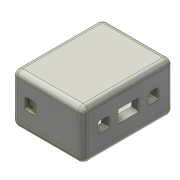
# Autodesk Inventor part: корпус емкость
Saved by Autodesk Inventor 2021 (Build 250183000, 183)
## iProperties
Created: 2023-02-13
Part Number: корпус емкость
Material: Типовые
Document SubType Name: Modeling
Designer: Tasya
Density: 1 g/cm^3
Appearance: Гладкий - слоновая кость
Author: Tasya
Autodesk Inventor part; units mm, degrees
ref_plane "YZ Plane" through (0, 0, 0) normal (1, 0, 0) x (0, 1, 0)
ref_plane "XZ Plane" through (0, 0, 0) normal (0, 1, 0) x (-1, 0, 0)
sketch "Эскиз1" plane through (0, 0, 0) normal (0, 1, 0) x (-1, 0, 0)
  line L0 (-20, 30) -> (20, 30)
  line L1 (20, 30) -> (20, -30)
  line L2 (20, -30) -> (-20, -30)
  line L3 (-20, -30) -> (-20, 30)
  line L4 (-20, 30) -> (20, -30) construction
  line L5 (20, 30) -> (-20, -30) construction
  point P0 (0, 0)
  dimension "d0" = 40
  dimension "d1" = 60
  constraints: 12 end point, 2 midpoint, 2 parallel, 1 horizontal, 1 perpendicular
  measures "d0" distance of L1.end L2.end
  measures "d1" distance of L0.end L1.end
extrude "Выдавливание1" add sketch "Эскиз1" along normal blind 30
shell "Оболочка1" thickness 3 outward yes removed faces 0
sketch "Эскиз22" plane through (-23, 0, -30) normal (1, 0, 0) x (0, 0, -1)
  line L0 (0, 0) -> (-60, 0) projected
  line L1 (0, 0) -> (0, 30) projected
  line L2 (0, 30) -> (-60, 30) projected
  line L3 (-60, 0) -> (-60, 30) projected
  line L4 (3, -3) -> (-63, -3) projected
  line L5 (-63, -3) -> (-63, 33) projected
  line L6 (3, 33) -> (-63, 33) projected
  line L7 (3, -3) -> (3, 33) projected
extrude "Выдавливание15" add sketch "Эскиз22" against normal blind 3 contours L0 L3 L2 L1 | L4 L5 L6 L7
sketch "Эскиз23" plane through (23, 0, 30) normal (-1, 0, 0) x (0, 0, 1)
  line L0 (0, 0) -> (-60, 0) projected
  line L1 (0, 0) -> (0, 30) projected
  line L2 (0, 30) -> (-60, 30) projected
  line L3 (-60, 0) -> (-60, 30) projected
  line L4 (3, -3) -> (-63, -3) projected
  line L5 (-63, -3) -> (-63, 33) projected
  line L6 (3, 33) -> (-63, 33) projected
  line L7 (3, -3) -> (3, 33) projected
  point P0 (-30, 0)
extrude "Выдавливание16" add sketch "Эскиз23" against normal blind 3 contours L0 L3 L2 L1 | L4 L5 L6 L7
fillet "Сопряжение1" radius 4 12 edges at (0, 33, 33) (0, -3, 33) (0, 33, -33) (0, -3, -33) (-26, 15, 33) (-26, 33, 0) (-26, -3, 0) (-26, 15, -33) (26, -3, 0) (26, 15, -33) (26, 33, 0) (26, 15, 33)
ref_plane "РабПлоскость1" through (0, 3, 0) normal (0, -1, 0) x (1, 0, 0)
split body "Разделение1" result two bodies by plane through (0, 3, 0) normal (0, -1, 0) first body at (7.333333, -2.5, 9.666667)
sketch "Эскиз24" plane through (-26, 3, 33) normal (0, -1, 0) x (1, 0, 0)
  line L0 (46, -63) -> (6, -63) construction
  line L1 (46, -3) -> (46, -63) construction
  line L2 (6, -3) -> (46, -3) construction
  line L3 (6, -63) -> (6, -3) construction
  line L4 (49, -3) -> (49, -63) construction
  line L5 (49, -63) -> (3, -63) construction
  line L6 (3, -63) -> (3, -3) construction
  line L7 (3, -3) -> (49, -3) construction
  line L8 (49, -3) -> (3, -63) construction
  line L9 (49, -63) -> (3, -3) construction
  line L10 (3, -3) -> (8, -8) construction
  line L11 (3, -3) -> (10.071068, -3) construction
  circle A0 centre (5.5, -5.5) radius 1.85 construction
  circle A1 centre (5.5, -5.5) radius 3.535534
  circle A2 centre (46.5, -5.5) radius 3.535534
  circle A3 centre (5.5, -60.5) radius 3.535534
  circle A4 centre (46.5, -60.5) radius 3.535534
  point P0 (26, -33)
  point P1 (44, -3)
  point P2 (3, -58)
  point P3 (44, -58)
  dimension "d168" = 45
  dimension "d169" = 3.7
  dimension "d170" = 2.5
  dimension "d171" = 46
  dimension "d172" = 60
  dimension "d175" = 41
  dimension "d178" = 55
  dimension "d230" = 3
  constraints: 16 end point, 3 horizontal, 3 midpoint, 3 vertical, 2 parallel, 1 centre point, 1 coincident, 1 collinear, 1 equal length, 1 perpendicular, 18 other
  measures "d168" angle of L10 L11
  measures "d169" diameter of A0
  measures "d170" distance from line of L2 A0.centre
  measures "d171" distance between parallel lines of L4 L6
  measures "d172" distance of L4.start L4.end
  measures "d175" distance of point (5.5, -5.5) point (46.5, -5.5)
  measures "d178" distance of point (5.5, -5.5) point (5.5, -60.5)
  measures "d230" distance between parallel lines of L4 L1
extrude "Выдавливание17" add sketch "Эскиз24" against normal up to next bodies 3
fillet "Сопряжение2" radius 2 16 edges at (-20, 30, 0) (0, 30, -30) (20, 30, 0) (0, 30, 30) (17.1459, 30, 26.382) (18, 16.5, 30) (20, 16.5, 24) (-20, 16.5, 24) (-18, 16.5, 30) (-17.1459, 30, 26.382) (-20, 16.5, -24) (-17.1459, 30, -26.382) (-18, 16.5, -30) (17.1459, 30, -26.382) (20, 16.5, -24) (18, 16.5, -30)
sketch "Эскиз25" plane through (-26, 3, 33) normal (0, -1, 0) x (1, 0, 0)
  line L0 (52, -4) -> (52, -62)
  line L1 (4, 0) -> (48, 0)
  line L2 (0, -62) -> (0, -4)
  line L3 (48, -66) -> (4, -66)
  arc A0 (7.096745, -8.654426) -> (9.021082, -5.180651) centre (5.5, -5.5) ccw
  line L4 (40.987094, -3) -> (11.012906, -3)
  arc A1 (42.978918, -5.180651) -> (44.903255, -8.654426) centre (46.5, -5.5) ccw
  arc A2 (46, -10.43884) -> (44.903255, -8.654426) centre (44, -10.43884) ccw
  line L5 (46, -55.56116) -> (46, -10.43884)
  arc A3 (44.903255, -57.345574) -> (46, -55.56116) centre (44, -55.56116) ccw
  arc A4 (44.903255, -57.345574) -> (42.978918, -60.819349) centre (46.5, -60.5) ccw
  line L6 (11.012906, -63) -> (40.987094, -63)
  arc A5 (9.021082, -60.819349) -> (7.096745, -57.345574) centre (5.5, -60.5) ccw
  arc A6 (6, -55.56116) -> (7.096745, -57.345574) centre (8, -55.56116) ccw
  line L7 (6, -10.43884) -> (6, -55.56116)
  arc A7 (7.096745, -8.654426) -> (6, -10.43884) centre (8, -10.43884) ccw
  arc A8 (0, -62) -> (4, -66) centre (4, -62) ccw
  arc A9 (48, -66) -> (52, -62) centre (48, -62) ccw
  arc A10 (52, -4) -> (48, 0) centre (48, -4) ccw
  arc A11 (4, 0) -> (0, -4) centre (4, -4) ccw
  arc A12 (11.012906, -3) -> (9.021082, -5.180651) centre (11.012906, -5) ccw
  arc A13 (42.978918, -5.180651) -> (40.987094, -3) centre (40.987094, -5) ccw
  arc A14 (40.987094, -63) -> (42.978918, -60.819349) centre (40.987094, -61) ccw
  arc A15 (9.021082, -60.819349) -> (11.012906, -63) centre (11.012906, -61) ccw
  point P0 (26, -33)
  point P1 (5.5, -5.5)
  point P2 (5.5, -60.5)
  constraints: 4 coincident
hole "Отверстие5" at (-20.5, 3, 27.5) at (20.5, 3, 27.5) at (-20.5, 3, -27.5) at (20.5, 3, -27.5) direction (0, 1, 0) diameter 3.7 depth 6 countersink diameter 4 countersink angle 90 bodies 3
sketch "Эскиз26" plane through (-26, 3, -33) normal (0, 1, 0) x (1, 0, 0)
  circle A0 centre (5.5, -5.5) radius 2
  circle A1 centre (5.5, -60.5) radius 2
  circle A2 centre (46.5, -60.5) radius 2
  circle A3 centre (46.5, -5.5) radius 2
  line L0 (52, -62) -> (52, -4)
  line L1 (4, -66) -> (48, -66)
  line L2 (0, -4) -> (0, -62)
  line L3 (48, 0) -> (4, 0)
  arc A4 (9.021082, -60.819349) -> (7.096745, -57.345574) centre (5.5, -60.5) ccw
  line L4 (40.987094, -63) -> (11.012906, -63)
  arc A5 (44.903255, -57.345574) -> (42.978918, -60.819349) centre (46.5, -60.5) ccw
  arc A6 (44.903255, -57.345574) -> (46, -55.56116) centre (44, -55.56116) ccw
  line L5 (46, -10.43884) -> (46, -55.56116)
  arc A7 (46, -10.43884) -> (44.903255, -8.654426) centre (44, -10.43884) ccw
  arc A8 (42.978918, -5.180651) -> (44.903255, -8.654426) centre (46.5, -5.5) ccw
  line L6 (11.012906, -3) -> (40.987094, -3)
  arc A9 (7.096745, -8.654426) -> (9.021082, -5.180651) centre (5.5, -5.5) ccw
  arc A10 (7.096745, -8.654426) -> (6, -10.43884) centre (8, -10.43884) ccw
  line L7 (6, -55.56116) -> (6, -10.43884)
  arc A11 (6, -55.56116) -> (7.096745, -57.345574) centre (8, -55.56116) ccw
  arc A12 (4, 0) -> (0, -4) centre (4, -4) ccw
  arc A13 (52, -4) -> (48, 0) centre (48, -4) ccw
  arc A14 (48, -66) -> (52, -62) centre (48, -62) ccw
  arc A15 (0, -62) -> (4, -66) centre (4, -62) ccw
  arc A16 (9.021082, -60.819349) -> (11.012906, -63) centre (11.012906, -61) ccw
  arc A17 (40.987094, -63) -> (42.978918, -60.819349) centre (40.987094, -61) ccw
  arc A18 (42.978918, -5.180651) -> (40.987094, -3) centre (40.987094, -5) ccw
  arc A19 (11.012906, -3) -> (9.021082, -5.180651) centre (11.012906, -5) ccw
  point P0 (26, -33)
extrude "Выдавливание18" add sketch "Эскиз26" against normal up to next contours A0 | A1 | A2 | A3 | A14 L1 A15 L2 A12 L3 A13 L0 bodies 2
fillet "Сопряжение3" radius 2 12 edges at (-20, 0, 0) (0, 0, 30) (19.7039, 0, 23.6084) (20, 0, 0) (19.7039, 0, -23.6084) (17.4073, 0, -25.7868) (17.4073, 0, 25.7868) (0, 0, -30) (-19.7039, 0, 23.6084) (-17.4073, 0, 25.7868) (-19.7039, 0, -23.6084) (-17.4073, 0, -25.7868)
sketch "Эскиз28" plane through (26, 0, 30) normal (1, 0, 0) x (0, 0, -1)
  line L0 (1, 3) -> (59, 3) projected
  line L1 (59, 29) -> (59, 3) projected
  line L2 (1, 29) -> (59, 29) projected
  line L3 (1, 3) -> (1, 29) projected
  line L4 (22.6, 20.5) -> (37.4, 20.5)
  line L5 (37.4, 20.5) -> (37.4, 11.5)
  line L6 (37.4, 11.5) -> (22.6, 11.5)
  line L7 (22.6, 11.5) -> (22.6, 20.5)
  line L8 (22.6, 20.5) -> (37.4, 11.5) construction
  line L9 (37.4, 20.5) -> (22.6, 11.5) construction
  line L10 (30, 0) -> (30, -11) construction
  line L11 (1, 3) -> (1, 29) construction
  line L12 (1, 16) -> (7, 16) construction
  point P0 (30, 16)
  point P1 (30, 16)
  point P2 (30, 16)
  dimension "d199" = 9
  dimension "d200" = 14.8
  constraints: 16 end point, 5 midpoint, 2 horizontal, 2 parallel, 2 point on line, 1 perpendicular, 1 vertical
  measures "d199" distance of L6.end L4.start
  measures "d200" distance of L5.end L6.end
extrude "Выдавливание20" cut sketch "Эскиз28" against normal blind 1.1 contours L4 L5 L6 L7 bodies 3
sketch "Эскиз29" plane through (24.9, 0, 30) normal (1, 0, 0) x (0, 0, -1)
  line L0 (37.4, 11.5) -> (22.6, 11.5) projected
  line L1 (37.4, 20.5) -> (37.4, 11.5) projected
  line L2 (22.6, 20.5) -> (37.4, 20.5) projected
  line L3 (22.6, 11.5) -> (22.6, 20.5) projected
  line L4 (21.7, 11.5) -> (38.3, 11.5)
  line L5 (38.3, 11.5) -> (38.3, 20.5)
  line L6 (38.3, 20.5) -> (21.7, 20.5)
  line L7 (21.7, 20.5) -> (21.7, 11.5)
  line L8 (21.7, 11.5) -> (38.3, 20.5) construction
  line L9 (38.3, 11.5) -> (21.7, 20.5) construction
  point P0 (30, 0)
  point P1 (30, 16)
  dimension "d203" = 0.9
  dimension "d204" = 0.9
  constraints: 12 end point, 2 collinear, 2 midpoint, 2 parallel, 1 horizontal, 1 perpendicular
  measures "d203" distance between parallel lines of L5 L1
  measures "d204" distance between parallel lines of L3 L7
extrude "Выдавливание21" cut sketch "Эскиз29" against normal blind 6 bodies 3
sketch "Эскиз30" plane through (-26, 0, -30) normal (-1, 0, 0) x (0, 0, 1)
  line L0 (1, 3) -> (59, 3) projected
  line L1 (59, 29) -> (59, 3) projected
  line L2 (1, 29) -> (59, 29) projected
  line L3 (1, 3) -> (1, 29) projected
  line L4 (1, 29) -> (1, 3) construction
  line L5 (1, 16) -> (59, 16) construction
  line L6 (30, 0) -> (30, 50) construction
  line L7 (22.5, 14) -> (7.5, 14)
  line L8 (7.5, 14) -> (7.5, 18)
  line L9 (7.5, 18) -> (22.5, 18)
  line L10 (22.5, 18) -> (22.5, 14)
  line L11 (22.5, 14) -> (7.5, 18) construction
  line L12 (7.5, 14) -> (22.5, 18) construction
  line L13 (52.5, 14) -> (37.5, 14)
  line L14 (37.5, 14) -> (37.5, 18)
  line L15 (37.5, 18) -> (52.5, 18)
  line L16 (52.5, 18) -> (52.5, 14)
  line L17 (52.5, 14) -> (37.5, 18) construction
  line L18 (37.5, 14) -> (52.5, 18) construction
  circle A0 centre (30, 16) radius 1.75 construction
  point P0 (15, 16)
  point P1 (45, 16)
  dimension "d207" = 4
  dimension "d208" = 15
  dimension "d209" = 3.5
  dimension "d210" = 15
  constraints: 28 end point, 7 midpoint, 4 parallel, 4 point on line, 2 horizontal, 2 perpendicular, 1 centre point, 1 collinear, 1 vertical, 1 other
  measures "d207" distance between parallel lines of L9 L7
  measures "d208" distance from line of L7.end L10
  measures "d209" diameter of A0
  measures "d210" distance from line of L13.end L10
extrude "Выдавливание22" add sketch "Эскиз30" along normal blind 4 contours L7 L8 L9 L10 | L13 L14 L15 L16 bodies 3
sketch "Эскиз31" plane through (-26, 0, -30) normal (-1, 0, 0) x (0, 0, 1)
  circle A0 centre (30, 16) radius 1.75 construction
  circle A1 centre (30, 16) radius 2.6
  point P0 (30, 0)
  dimension "d213" = 5.2
  constraints: 1 centre point, 1 coincident
  measures "d213" diameter of A1
extrude "Выдавливание23" cut sketch "Эскиз31" against normal blind 1.7 bodies 3
sketch "Эскиз33" plane through (-22, 29, 33) normal (0, 0, 1) x (1, 0, 0)
  line L0 (0, -26) -> (44, -26) projected
  line L1 (44, 0) -> (44, -26) projected
  line L2 (0, 0) -> (44, 0) projected
  line L3 (0, -26) -> (0, 0) projected
  line L4 (44, -26) -> (44, 0) construction
  line L5 (44, -13) -> (0, -13) construction
  line L6 (0, 0) -> (0, -26) construction
  line L7 (6, -9.5) -> (13, -9.5)
  line L8 (13, -9.5) -> (13, -16.5)
  line L9 (13, -16.5) -> (6, -16.5)
  line L10 (6, -16.5) -> (6, -9.5)
  line L11 (6, -9.5) -> (13, -16.5) construction
  line L12 (13, -9.5) -> (6, -16.5) construction
  point P0 (22, -29)
  point P1 (9.5, -13)
  dimension "d220" = 7
  dimension "d221" = 7
  dimension "d222" = 6
  constraints: 14 end point, 4 midpoint, 2 parallel, 1 horizontal, 1 perpendicular, 1 point on line
  measures "d220" distance of L8.end L9.end
  measures "d221" distance of L7.end L8.end
  measures "d222" distance between parallel lines of L3 L10
extrude "Выдавливание25" cut sketch "Эскиз33" against normal blind 6 contours L7 L8 L9 L10 bodies 3
sketch "Эскиз34" plane through (0, -3, 0) normal (0, -1, 0) x (1, 0, 0)
  line L0 (18, -22.56116) -> (18, 22.56116)
  line L1 (7.5, 21.5) -> (7.5, -21.343284) construction
  line L2 (7.5, -21.343284) -> (-5.111414, -21.343284) construction
  line L3 (-5.111414, -21.343284) -> (-5.111414, 21.5) construction
  line L4 (-5.111414, 21.5) -> (7.5, 21.5) construction
  line L5 (22, 29) -> (22, -29)
  line L6 (-22, -29) -> (-22, 29)
  line L7 (-14.987094, 30) -> (14.987094, 30)
  line L8 (-22, 29) -> (22, 29)
  line L9 (22, -29) -> (-22, -29)
  line L10 (-2.710696, 21.56483) -> (7.289304, 18.193679)
  line L11 (7.289304, 18.193679) -> (7.289304, 16.556726)
  line L12 (7.289304, 16.556726) -> (-2.710696, 13.185575)
  line L13 (-2.710696, 13.185575) -> (-2.710696, 14.58752)
  line L14 (-2.710696, 14.58752) -> (0.08509, 15.495138)
  line L15 (0.08509, 15.495138) -> (0.08509, 19.311994)
  line L16 (0.08509, 19.311994) -> (-2.710696, 20.219611)
  line L17 (-2.710696, 20.219611) -> (-2.710696, 21.56483)
  line L18 (1.219611, 15.859806) -> (5.927877, 17.407618)
  line L19 (5.927877, 17.407618) -> (1.219611, 18.947326)
  line L20 (1.219611, 18.947326) -> (1.219611, 15.859806)
  spline S0 degree 2 poles (0.360616, 5.454619) (-0.384927, 5.454619) (-1.527552, 6.02188) (-1.900324, 6.491896) knots 0 0 0 1 2 2 2
  spline S1 degree 2 poles (-1.900324, 6.491896) (-2.337925, 7.059157) (-2.710696, 8.34765) (-2.710696, 9.36872) knots 0 0 0 1 2 2 2
  line L21 (-2.710696, 9.36872) -> (-2.710696, 12.237439)
  line L22 (-2.710696, 12.237439) -> (7.289304, 12.237439)
  line L23 (7.289304, 12.237439) -> (7.289304, 9.58752)
  spline S2 degree 2 poles (7.289304, 9.58752) (7.289304, 8.517828) (7.15154, 7.448136) (6.884117, 6.961912) knots 0 0 0 1 2 2 2
  spline S3 degree 2 poles (6.884117, 6.961912) (6.600487, 6.418963) (5.668558, 5.924635) (5.036467, 5.924635) knots 0 0 0 1 2 2 2
  spline S4 degree 2 poles (5.036467, 5.924635) (4.331443, 5.924635) (3.213129, 6.670178) (2.897083, 7.32658) knots 0 0 0 1 2 2 2
  line L24 (2.897083, 7.32658) -> (2.848461, 7.32658)
  spline S5 degree 2 poles (2.848461, 7.32658) (2.605349, 6.43517) (1.316856, 5.454619) (0.360616, 5.454619) knots 0 0 0 1 2 2 2
  spline S6 degree 2 poles (0.30389, 6.840357) (0.871151, 6.840357) (1.600487, 7.164506) (1.859806, 7.650729) knots 0 0 0 1 2 2 2
  spline S7 degree 2 poles (1.859806, 7.650729) (2.021881, 7.966775) (2.119125, 8.712318) (2.119125, 9.401135) knots 0 0 0 1 2 2 2
  line L25 (2.119125, 9.401135) -> (2.119125, 10.908428)
  line L26 (2.119125, 10.908428) -> (-1.576175, 10.908428)
  line L27 (-1.576175, 10.908428) -> (-1.576175, 9.830632)
  spline S8 degree 2 poles (-1.576175, 9.830632) (-1.576175, 8.955429) (-1.4141, 7.950567) (-1.154781, 7.561588) knots 0 0 0 1 2 2 2
  spline S9 degree 2 poles (-1.154781, 7.561588) (-0.887358, 7.188817) (-0.222852, 6.840357) (0.30389, 6.840357) knots 0 0 0 1 2 2 2
  spline S10 degree 2 poles (4.850081, 7.310373) (5.206646, 7.310373) (5.741492, 7.553485) (5.895462, 7.820908) knots 0 0 0 1 2 2 2
  spline S11 degree 2 poles (5.895462, 7.820908) (6.073744, 8.145057) (6.154782, 8.931118) (6.154782, 9.636143) knots 0 0 0 1 2 2 2
  line L28 (6.154782, 9.636143) -> (6.154782, 10.908428)
  line L29 (6.154782, 10.908428) -> (3.229336, 10.908428)
  line L30 (3.229336, 10.908428) -> (3.229336, 9.401135)
  spline S12 degree 2 poles (3.229336, 9.401135) (3.229336, 8.777147) (3.358996, 8.185575) (3.561589, 7.86953) knots 0 0 0 1 2 2 2
  spline S13 degree 2 poles (3.561589, 7.86953) (3.756078, 7.561588) (4.380065, 7.310373) (4.850081, 7.310373) knots 0 0 0 1 2 2 2
  line L31 (-2.710696, -3.054295) -> (-2.710696, -1.725284)
  line L32 (-2.710696, -1.725284) -> (5.230957, -1.725284)
  line L33 (5.230957, -1.725284) -> (-2.710696, 2.788493)
  line L34 (-2.710696, 2.788493) -> (-2.710696, 4.133712)
  line L35 (-2.710696, 4.133712) -> (7.289304, 4.133712)
  line L36 (7.289304, 4.133712) -> (7.289304, 2.8047)
  line L37 (7.289304, 2.8047) -> (-0.52269, 2.8047)
  line L38 (-0.52269, 2.8047) -> (7.289304, -1.644246)
  line L39 (7.289304, -1.644246) -> (7.289304, -3.054295)
  line L40 (7.289304, -3.054295) -> (-2.710696, -3.054295)
  spline S14 degree 2 poles (6.146678, -12.154781) (5.482172, -12.722042) (3.537278, -13.354133) (2.289304, -13.354133) knots 0 0 0 1 2 2 2
  spline S15 degree 2 poles (2.289304, -13.354133) (1.073744, -13.354133) (-0.895461, -12.73825) (-1.559967, -12.154781) knots 0 0 0 1 2 2 2
  spline S16 degree 2 poles (-1.559967, -12.154781) (-2.256888, -11.538898) (-2.921393, -9.910049) (-2.921393, -8.929498) knots 0 0 0 1 2 2 2
  spline S17 degree 2 poles (-2.921393, -8.929498) (-2.921393, -7.916532) (-2.232577, -6.295786) (-1.559967, -5.704214) knots 0 0 0 1 2 2 2
  spline S18 degree 2 poles (-1.559967, -5.704214) (-0.895461, -5.128849) (1.057537, -4.512966) (2.289304, -4.512966) knots 0 0 0 1 2 2 2
  spline S19 degree 2 poles (2.289304, -4.512966) (3.545381, -4.512966) (5.457861, -5.136953) (6.146678, -5.712318) knots 0 0 0 1 2 2 2
  spline S20 degree 2 poles (6.146678, -5.712318) (6.811184, -6.295786) (7.5, -7.924635) (7.5, -8.929498) knots 0 0 0 1 2 2 2
  spline S21 degree 2 poles (7.5, -8.929498) (7.5, -9.950567) (6.786872, -11.58752) (6.146678, -12.154781) knots 0 0 0 1 2 2 2
  spline S22 degree 2 poles (2.289304, -11.968395) (3.277958, -11.968395) (4.809563, -11.538898) (5.311994, -11.149919) knots 0 0 0 1 2 2 2
  spline S23 degree 2 poles (5.311994, -11.149919) (5.830633, -10.752836) (6.349271, -9.634522) (6.349271, -8.937601) knots 0 0 0 1 2 2 2
  spline S24 degree 2 poles (6.349271, -8.937601) (6.349271, -8.21637) (5.84684, -7.13047) (5.311994, -6.71718) knots 0 0 0 1 2 2 2
  spline S25 degree 2 poles (5.311994, -6.71718) (4.801459, -6.320097) (3.261751, -5.898703) (2.289304, -5.898703) knots 0 0 0 1 2 2 2
  spline S26 degree 2 poles (2.289304, -5.898703) (0.320098, -5.898703) (-1.770664, -7.551864) (-1.770664, -8.937601) knots 0 0 0 1 2 2 2
  spline S27 degree 2 poles (-1.770664, -8.937601) (-1.770664, -10.323339) (0.320098, -11.968395) (2.289304, -11.968395) knots 0 0 0 1 2 2 2
  spline S28 degree 2 poles (4.274717, -21.133712) (3.626419, -21.133712) (2.459482, -20.671799) (2.054295, -20.258509) knots 0 0 0 1 2 2 2
  spline S29 degree 2 poles (2.054295, -20.258509) (1.543761, -19.73987) (1.017018, -18.337925) (1.017018, -17.268233) knots 0 0 0 1 2 2 2
  line L41 (1.017018, -17.268233) -> (1.017018, -16.141815)
  line L42 (1.017018, -16.141815) -> (-2.710696, -16.141815)
  line L43 (-2.710696, -16.141815) -> (-2.710696, -14.812804)
  line L44 (-2.710696, -14.812804) -> (7.289304, -14.812804)
  line L45 (7.289304, -14.812804) -> (7.289304, -17.324959)
  spline S30 degree 2 poles (7.289304, -17.324959) (7.289304, -18.21637) (6.997569, -19.464344) (6.665317, -19.942464) knots 0 0 0 1 2 2 2
  spline S31 degree 2 poles (6.665317, -19.942464) (6.284441, -20.501621) (5.109401, -21.133712) (4.274717, -21.133712) knots 0 0 0 1 2 2 2
  spline S32 degree 2 poles (4.234198, -19.747974) (4.752837, -19.747974) (5.514587, -19.39141) (5.757699, -19.026742) knots 0 0 0 1 2 2 2
  spline S33 degree 2 poles (5.757699, -19.026742) (5.968396, -18.710697) (6.138574, -17.867909) (6.138574, -17.243922) knots 0 0 0 1 2 2 2
  line L46 (6.138574, -17.243922) -> (6.138574, -16.141815)
  line L47 (6.138574, -16.141815) -> (2.15154, -16.141815)
  line L48 (2.15154, -16.141815) -> (2.15154, -17.049433)
  spline S34 degree 2 poles (2.15154, -17.049433) (2.15154, -17.859806) (2.410859, -18.856564) (2.751216, -19.180713) knots 0 0 0 1 2 2 2
  spline S35 degree 2 poles (2.751216, -19.180713) (3.051054, -19.480551) (3.756078, -19.747974) (4.234198, -19.747974) knots 0 0 0 1 2 2 2
  point P0 (0, 0)
  point P1 (19.5, 25.855163)
  point P2 (19.5, -25.855163)
  point P3 (-19.5, -25.855163)
  point P4 (-19.5, 25.855163)
  point P5 (-17.5, 30)
  point P6 (17.5, 30)
  point P7 (-17.2, 29)
  point P8 (17.2, 29)
  point P9 (17.2, -29)
  point P10 (-17.2, -29)
  dimension "d226" = 14.5
  dimension "d227" = 7.5
  constraints: 4 other
  measures "d227" distance between parallel lines of L8 L4
extrude "Выдавливание26" cut sketch "Эскиз34" against normal blind 0.5 contours L10 L11 L12 L13 L14 L15 L16 L17 | S0 S1 L21 L22 L23 S2 S3 S4 L24 S5 | L31 L32 L33 L34 L35 L36 L37 L38 L39 L40 | S14 S15 S16 S17 S18 S19 S20 S21 | S28 S29 L41 L42 L43 L44 L45 S30 S31 bodies 2
sketch "Эскиз35" plane through (0, -3, 0) normal (0, -1, 0) x (1, 0, 0)
  arc A0 (-26, -29) -> (-22, -33) centre (-22, -29) ccw
  line L0 (-26, -29) -> (-26, 29)
  arc A1 (-22, 33) -> (-26, 29) centre (-22, 29) ccw
  line L1 (-22, 33) -> (22, 33)
  arc A2 (26, 29) -> (22, 33) centre (22, 29) ccw
  line L2 (26, 29) -> (26, -29)
  arc A3 (22, -33) -> (26, -29) centre (22, -29) ccw
  line L3 (22, -33) -> (-22, -33)
  arc A4 (-20, -22.56116) -> (-18.903255, -24.345574) centre (-18, -22.56116) ccw
  arc A5 (-16.978918, -27.819349) -> (-18.903255, -24.345574) centre (-20.5, -27.5) ccw
  arc A6 (-16.978918, -27.819349) -> (-14.987094, -30) centre (-14.987094, -28) ccw
  line L4 (-14.987094, -30) -> (14.987094, -30)
  arc A7 (14.987094, -30) -> (16.978918, -27.819349) centre (14.987094, -28) ccw
  arc A8 (18.903255, -24.345574) -> (16.978918, -27.819349) centre (20.5, -27.5) ccw
  arc A9 (18.903255, -24.345574) -> (20, -22.56116) centre (18, -22.56116) ccw
  line L5 (20, -22.56116) -> (20, 22.56116)
  arc A10 (20, 22.56116) -> (18.903255, 24.345574) centre (18, 22.56116) ccw
  arc A11 (16.978918, 27.819349) -> (18.903255, 24.345574) centre (20.5, 27.5) ccw
  arc A12 (16.978918, 27.819349) -> (14.987094, 30) centre (14.987094, 28) ccw
  line L6 (14.987094, 30) -> (-14.987094, 30)
  arc A13 (-14.987094, 30) -> (-16.978918, 27.819349) centre (-14.987094, 28) ccw
  arc A14 (-18.903255, 24.345574) -> (-16.978918, 27.819349) centre (-20.5, 27.5) ccw
  arc A15 (-18.903255, 24.345574) -> (-20, 22.56116) centre (-18, 22.56116) ccw
  line L7 (-20, 22.56116) -> (-20, -22.56116)
  point P0 (0, 0)
  constraints: 4 coincident
hole "Отверстие6" at (20.5, -3, 27.5) at (-20.5, -3, 27.5) at (-20.5, -3, -27.5) at (20.5, -3, -27.5) direction (0, 1, 0) diameter 3.4 end through all countersink diameter 6.6 countersink angle 90 bodies 2 clearance for "с потайной головкой ГОСТ 12876-67" size "M3" standard "ГОСТ"
sketch "Эскиз36" plane through (26, 0, 30) normal (1, 0, 0) x (0, 0, -1)
  line L0 (37.4, 20.5) -> (37.4, 11.5)
  line L1 (37.4, 11.5) -> (22.6, 11.5)
  line L2 (22.6, 11.5) -> (22.6, 20.5)
  line L3 (22.6, 20.5) -> (37.4, 20.5)
  line L4 (1, 3) -> (59, 3)
  line L5 (59, 29) -> (59, 3)
  line L6 (1, 29) -> (59, 29)
  line L7 (1, 3) -> (1, 29)
  line L8 (1, 3) -> (1, 29) construction
  line L9 (1, 16) -> (59, 16) construction
  line L10 (52.56116, 30) -> (7.43884, 30) construction
  line L11 (30, 30) -> (30, 0) construction
  line L12 (8.6, 12.5) -> (15.6, 12.5)
  line L13 (15.6, 12.5) -> (15.6, 19.5)
  line L14 (15.6, 19.5) -> (8.6, 19.5)
  line L15 (8.6, 19.5) -> (8.6, 12.5)
  line L16 (8.6, 12.5) -> (15.6, 19.5) construction
  line L17 (15.6, 12.5) -> (8.6, 19.5) construction
  line L18 (59, 3) -> (59, 29)
  line L19 (51.4, 12.5) -> (44.4, 12.5)
  line L20 (44.4, 12.5) -> (44.4, 19.5)
  line L21 (44.4, 19.5) -> (51.4, 19.5)
  line L22 (51.4, 19.5) -> (51.4, 12.5)
  line L23 (51.4, 12.5) -> (44.4, 19.5) construction
  line L24 (44.4, 12.5) -> (51.4, 19.5) construction
  point P0 (12.1, 16)
  point P1 (47.9, 16)
  dimension "d238" = 7
  dimension "d239" = 7
  dimension "d240" = 7
  constraints: 30 end point, 7 midpoint, 5 symmetric about line, 2 parallel, 1 horizontal, 1 perpendicular, 1 point on line, 1 vertical
  measures "d238" distance of L14.end L13.end
  measures "d239" distance of L13.end L12.end
  measures "d240" distance from line of L1.end L13
extrude "Выдавливание27" cut sketch "Эскиз36" against normal blind 6 contours L15 L14 L13 L12 | L19 L20 L21 L22 bodies 3
fillet "Сопряжение6" radius 1 38 edges at (-9, 19.5, 31.5) (-9, 16, 33) (-12.5, 12.5, 33) (-9, 16, 30) (-9, 12.5, 31.5) (-12.5, 19.5, 33) (-11.9935, 19.5, 30) (-16, 19.5, 31.3623) (-16, 16, 33) (-16, 12.5, 31.3623) (-15.5119, 19.5, 29.9299) (-16, 16, 29.7245) (-15.5119, 12.5, 29.9299) (-11.9935, 12.5, 30) (26, 19.5, 17.9) (20, 19.5, 17.9) (23, 19.5, 21.4) (23, 19.5, 14.4) (26, 16, 14.4) (26, 16, 21.4) (20, 16, 21.4) (20, 16, 14.4) (23, 12.5, 14.4) (23, 12.5, 21.4) (26, 12.5, 17.9) (20, 12.5, 17.9) (23, 19.5, -14.4) (26, 19.5, -17.9) (26, 16, -14.4) (20, 19.5, -17.9) (23, 19.5, -21.4) (26, 16, -21.4) (20, 16, -21.4) (20, 16, -14.4) (23, 12.5, -14.4) (20, 12.5, -17.9) (26, 12.5, -17.9) (23, 12.5, -21.4)
sketch "Эскиз39" plane through (-14.987094, 30, -28) normal (0, -1, 0) x (1, 0, 0)
  line L0 (29.974187, 0) -> (0, 0)
  arc A0 (32.987094, 5.43884) -> (29.974187, 0) centre (35.487094, 0.5) ccw
  line L1 (32.987094, 50.56116) -> (32.987094, 5.43884)
  arc A1 (29.974187, 56) -> (32.987094, 50.56116) centre (35.487094, 55.5) ccw
  line L2 (0, 56) -> (29.974187, 56)
  arc A2 (-3.012906, 50.56116) -> (0, 56) centre (-5.512906, 55.5) ccw
  line L3 (-3.012906, 5.43884) -> (-3.012906, 50.56116)
  arc A3 (0, 0) -> (-3.012906, 5.43884) centre (-5.512906, 0.5) ccw
  line L4 (1.987094, 53) -> (27.987094, 53) construction
  line L5 (27.987094, 53) -> (27.987094, 3) construction
  line L6 (27.987094, 3) -> (1.987094, 3) construction
  line L7 (1.987094, 3) -> (1.987094, 53) construction
  line L8 (1.987094, 53) -> (27.987094, 3) construction
  line L9 (27.987094, 53) -> (1.987094, 3) construction
  circle A4 centre (30.487094, 46) radius 2.5
  line L10 (14.987094, 28) -> (14.987094, 20) construction
  circle A5 centre (-0.512906, 46) radius 2.5
  line L11 (30.487094, 48.5) -> (-0.512906, 48.5)
  line L12 (-0.512906, 43.5) -> (30.487094, 43.5)
  line L13 (14.987094, 28) -> (21, 28) construction
  dimension "d254" = 26
  dimension "d255" = 50
  dimension "d256" = 5
  dimension "d257" = 18
  constraints: 20 end point, 5 tangent, 4 point on circle, 2 centre point, 2 horizontal, 2 midpoint, 2 parallel, 1 perpendicular, 1 symmetric about line, 1 vertical, 1 other
  measures "d254" distance of L5.end L6.end
  measures "d255" distance of L4.end L5.end
  measures "d256" diameter of A4
  measures "d257" vertical distance of L10.start A4.centre
extrude "Выдавливание30" add sketch "Эскиз39" along normal blind 3 contours A4 | A5 | A4 L12 A5 L11 bodies 3
mirror "Зеркальное отражение1" about plane through (0, 0, 0) normal (0, 0, 1) of "Выдавливание30" bodies 3
sketch "Эскиз40" plane through (-14.987094, 27, -28) normal (0, -1, 0) x (1, 0, 0)
  arc A0 (30.487094, 43.5) -> (30.487094, 48.5) centre (30.487094, 46) ccw
  line L0 (30.487094, 48.5) -> (-0.512906, 48.5)
  arc A1 (-0.512906, 48.5) -> (-0.512906, 43.5) centre (-0.512906, 46) ccw
  line L1 (-0.512906, 43.5) -> (30.487094, 43.5)
  arc A2 (30.487094, 7.5) -> (30.487094, 12.5) centre (30.487094, 10) ccw
  line L2 (-0.512906, 12.5) -> (30.487094, 12.5)
  arc A3 (-0.512906, 12.5) -> (-0.512906, 7.5) centre (-0.512906, 10) ccw
  line L3 (30.487094, 7.5) -> (-0.512906, 7.5)
  point P0 (14.987094, 28)
  constraints: 4 coincident
hole "Отверстие7" at (15.5, 27, -18) at (-15.5, 27, -18) direction (0, 1, 0) diameter 2.4 depth 3 countersink diameter 3 countersink angle 90 bodies 3
sketch "Эскиз41" plane through (-14.987094, 27, -28) normal (0, -1, 0) x (1, 0, 0)
  line L0 (1.987094, 6) -> (27.987094, 6) construction
  line L1 (27.987094, 6) -> (27.987094, 50) construction
  line L2 (27.987094, 50) -> (1.987094, 50) construction
  line L3 (1.987094, 50) -> (1.987094, 6) construction
  line L4 (1.987094, 6) -> (27.987094, 50) construction
  line L5 (27.987094, 6) -> (1.987094, 50) construction
  arc A0 (30.487094, 43.5) -> (30.487094, 48.5) centre (30.487094, 46) ccw
  line L6 (30.487094, 48.5) -> (-0.512906, 48.5)
  arc A1 (-0.512906, 48.5) -> (-0.512906, 43.5) centre (-0.512906, 46) ccw
  line L7 (-0.512906, 43.5) -> (30.487094, 43.5)
  line L8 (27.987094, 48.5) -> (27.987094, 43.5)
  line L9 (30.487094, 48.5) -> (-0.512906, 48.5)
  line L10 (1.987094, 48.5) -> (1.987094, 43.5)
  point P0 (14.987094, 28)
  dimension "d267" = 26
  constraints: 16 end point, 8 point on line, 2 midpoint, 2 parallel, 1 horizontal, 1 perpendicular
  measures "d267" distance of L2.end L1.end
extrude "Выдавливание31" cut sketch "Эскиз41" against normal blind 3 contours L7 L8 L6 A0 | L7 A1 L6 L10 bodies 3
fillet "Сопряжение7" radius 2 4 edges at (13, 28.5, 15.5) (13, 28.5, 20.5) (-13, 28.5, 15.5) (-13, 28.5, 20.5)
